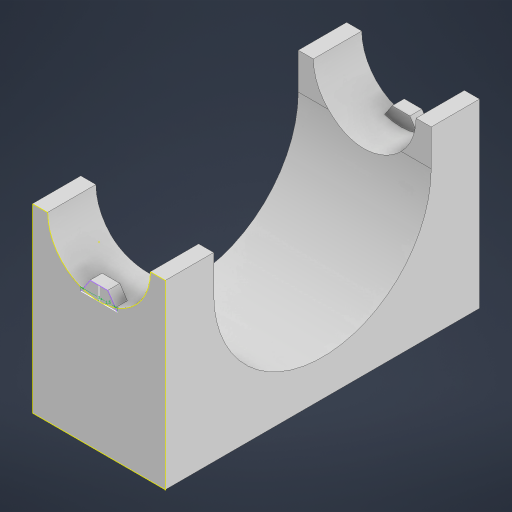
# Autodesk Inventor part: Part5
Saved by Autodesk Inventor 2023 (Build 270158030, 158C)
## iProperties
Created: 2023-02-06
Part Number: Part5
Material: Generic
Document SubType Name: Modeling
Designer: Monster
Density: 1 g/cm^3
Appearance: Default
Author: Monster
Autodesk Inventor part; units mm, degrees
ref_plane "YZ Plane" through (0, 0, 0) normal (1, 0, 0) x (0, 1, 0)
ref_plane "XZ Plane" through (0, 0, 0) normal (0, 1, 0) x (-1, 0, 0)
ref_plane "XY Plane" through (0, 0, 0) normal (0, 0, 1) x (1, 0, 0)
sketch "Sketch2" plane through (0, 0, 0) normal (0, 1, 0) x (-1, 0, 0)
  line L0 (0, 0) -> (0, -26)
  line L1 (0, -26) -> (11, -26)
  line L2 (11, -26) -> (11, 0)
  line L3 (11, 0) -> (0, 0)
  dimension "d2" = 26
  dimension "d3" = 11
  constraints: 8 end point, 3 perpendicular, 1 vertical
  measures "d2" distance of L0.start L0.end
  measures "d3" distance of L0.end L1.end
extrude "Extrusion1" add sketch "Sketch2" along normal blind 15
sketch "Sketch3" plane through (-11, 0, 0) normal (0, 0, 1) x (1, 0, 0)
  line L0 (0, 0) -> (11, 0) projected
  line L1 (11, 0) -> (11, 15) projected
  line L2 (0, 15) -> (11, 15) projected
  line L3 (0, 0) -> (0, 15) projected
  line L4 (11, 15) -> (0, 15) projected
  circle A0 centre (5.5, 15) radius 4.25
  point P0 (9.75, 15)
  point P1 (1.25, 15)
  dimension "d6" = 8.5
  constraints: 1 centre point, 1 midpoint
  measures "d6" diameter of A0
extrude "Extrusion2" cut sketch "Sketch3" against normal blind 32.25 contours L2 A0 picked at (4.2044, 14.0026)
sketch "Sketch4" plane through (0, 0, 0) normal (1, 0, 0) x (0, 0, -1)
  line L0 (0, 0) -> (26, 0) projected
  line L1 (26, 0) -> (26, 15) projected
  line L2 (0, 15) -> (26, 15) projected
  line L3 (0, 0) -> (0, 15) projected
  line L4 (0, 15) -> (4, 15)
  line L5 (0, 15) -> (26, 15) projected
  line L6 (26, 15) -> (22, 15)
  line L7 (22, 15) -> (22, 12)
  line L8 (0, 10.75) -> (26, 10.75) projected
  line L9 (22, 12) -> (4, 12)
  line L10 (4, 12) -> (4, 15)
  line L11 (26, 0) -> (0, 0) projected
  line L12 (13, 0) -> (13, 3)
  arc A0 (4, 12) -> (22, 12) centre (13, 12) ccw
  dimension "d9" = 4
  dimension "d10" = 4
  dimension "d11" = 3
  dimension "d12" = 3
  constraints: 12 end point, 3 perpendicular, 3 point on circle, 2 point on line, 1 centre point, 1 midpoint, 1 vertical
  measures "d9" distance of L2.start L4.end
  measures "d10" distance of L1.end L6.end
  measures "d11" distance of L6.end L7.end
  measures "d12" distance of L12.start L12.end
extrude "Extrusion3" cut sketch "Sketch4" against normal blind 32.25 contours A0 L8 | A0 L9 L8 | L2 L7 L9 L10
sketch "Sketch5" plane through (-11, 0, 0) normal (0, 0, 1) x (1, 0, 0)
  arc A0 (1.25, 15) -> (9.75, 15) centre (5.5, 15) ccw projected
  line L0 (0, 15) -> (1.25, 15) projected
  line L1 (0, 0) -> (0, 15) projected
  line L2 (0, 0) -> (11, 0) projected
  line L3 (11, 0) -> (11, 15) projected
  line L4 (9.75, 15) -> (11, 15) projected
  arc A1 (1.25, 15) -> (9.75, 15) centre (5.5, 15) ccw projected
  line L5 (5.5, 10.75) -> (7, 10.75)
  line L6 (7, 10.75) -> (4, 10.75)
  line L7 (4, 10.75) -> (4.7672, 11.9025)
  line L8 (4.7672, 11.9025) -> (5.5, 11.9025)
  line L9 (5.5, 11.9025) -> (5.5, 10.75)
  line L10 (7, 10.75) -> (6.2328, 11.9025)
  line L11 (6.2328, 11.9025) -> (5.5, 11.9025)
  arc A2 (1.25, 15) -> (9.75, 15) centre (5.5, 15) ccw projected
  line L12 (11, 15) -> (9.75, 15) projected
  line L13 (11, 0) -> (11, 15) projected
  line L14 (11, 0) -> (0, 0) projected
  line L15 (0, 0) -> (0, 15) projected
  line L16 (1.25, 15) -> (0, 15) projected
  line L17 (5.5, 10.75) -> (4, 10.75)
  line L18 (4, 10.75) -> (4.7672, 11.9025)
  line L19 (6.2328, 11.9025) -> (6.1284, 11.9025)
  line L20 (6.2328, 11.9025) -> (4.7672, 11.9025)
  line L21 (6.2328, 11.9025) -> (7, 10.75)
  line L22 (7, 10.75) -> (4, 10.75)
  arc A3 (1.25, 15) -> (9.75, 15) centre (5.5, 15) ccw projected
  line L23 (11, 15) -> (9.75, 15) projected
  line L24 (11, 0) -> (11, 15) projected
  line L25 (11, 0) -> (0, 0) projected
  line L26 (0, 0) -> (0, 15) projected
  line L27 (1.25, 15) -> (0, 15) projected
  arc A4 (1.25, 15) -> (9.75, 15) centre (5.5, 15) ccw projected
  line L28 (11, 15) -> (9.75, 15) projected
  line L29 (11, 0) -> (11, 15) projected
  line L30 (11, 0) -> (0, 0) projected
  line L31 (0, 0) -> (0, 15) projected
  line L32 (1.25, 15) -> (0, 15) projected
  point P0 (4.1472, 10.9711)
  point P1 (6.8528, 10.9711)
  dimension "d15" = 1.5
  dimension "d16" = 3
  constraints: 26 end point, 3 collinear, 3 point on circle, 2 point on line, 1 horizontal, 1 midpoint, 1 parallel, 1 symmetric about line, 1 tangent
  measures "d15" distance of L5.start L5.end
  measures "d16" distance of L5.end L6.end
extrude "Extrusion4" add sketch "Sketch5" against normal blind 1 contours L7 L8 L9 A0 | L9 L11 L10 A0
sketch "Sketch6" plane through (0, 0, -26) normal (0, 0, -1) x (-1, 0, 0)
  arc A0 (1.25, 15) -> (9.75, 15) centre (5.5, 15) ccw projected
  line L0 (0, 15) -> (1.25, 15) projected
  line L1 (0, 0) -> (0, 15) projected
  line L2 (0, 0) -> (11, 0) projected
  line L3 (11, 0) -> (11, 15) projected
  line L4 (9.75, 15) -> (11, 15) projected
  arc A1 (4.1472, 10.9711) -> (6.8528, 10.9711) centre (5.5, 15) ccw projected
  line L5 (5.5, 10.75) -> (7, 10.75)
  line L6 (4.7672, 11.9025) -> (6.2328, 11.9025) projected
  line L7 (7, 10.75) -> (6.2328, 11.9025)
  line L8 (6.2328, 11.9025) -> (4.7672, 11.9025)
  line L9 (4.7672, 11.9025) -> (4, 10.75)
  line L10 (4.7672, 11.9025) -> (4.1472, 10.9711) projected
  line L11 (4, 10.75) -> (5.5, 10.75)
  point P0 (0, 0)
  point P1 (6.8528, 10.9711)
  dimension "d19" = 1.5
  constraints: 10 end point, 3 collinear, 2 point on circle, 2 tangent, 1 horizontal, 1 point on line
  measures "d19" distance of L5.start L5.end
extrude "Extrusion5" add sketch "Sketch6" against normal blind 1 contours L9 L6 L7 A0
body "Solid1"
